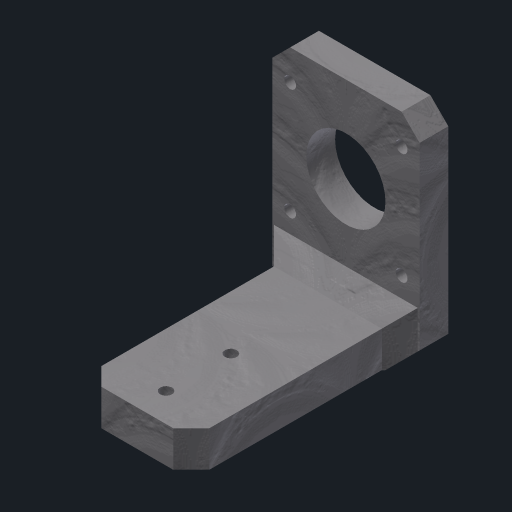
# Autodesk Inventor part: SOPORTE_NEMA_2
Saved by Autodesk Inventor 2024.3 (Build 283343000, 343)
## iProperties
Created: 2024-07-10
Part Number: SOPORTE_NEMA_2
Material: Steel, Mild, Welded
Document SubType Name: Modeling
Designer: Niler
Density: 7.85 g/cm^3
Appearance: Weld - Steel Mild
Author: Niler
Autodesk Inventor part; units mm, degrees
ref_plane "YZ Plane" through (0, 0, 0) normal (1, 0, 0) x (0, 1, 0)
ref_plane "XZ Plane" through (0, 0, 0) normal (0, 1, 0) x (-1, 0, 0)
ref_plane "XY Plane" through (0, 0, 0) normal (0, 0, 1) x (1, 0, 0)
sketch "Sketch1" plane through (0, 0, 0) normal (0, 1, 0) x (-1, 0, 0)
  line L0 (-15, 0) -> (15, 0)
  line L1 (15, 0) -> (15, -66)
  line L2 (15, -66) -> (-15, -66)
  line L3 (-15, -66) -> (-15, 0)
  circle A0 centre (0, -8) radius 1.65
  circle A1 centre (0, -26) radius 1.65
  point P0 (0, 0)
  point P1 (0, 0)
  dimension "d0" = 66
  dimension "d1" = 30
  dimension "d2" = 3.3
  dimension "d3" = 3.3
  dimension "d4" = 18
  dimension "d5" = 8
  constraints: 8 end point, 2 centre point, 2 coincident, 2 parallel, 1 horizontal, 1 midpoint, 1 perpendicular, 1 vertical alignment
  measures "d0" distance between parallel lines of L0 L2
  measures "d1" distance of L0.start L0.end
  measures "d2" diameter of A0
  measures "d3" diameter of A1
  measures "d4" distance of A1.centre A0.centre
  measures "d5" distance from line of L0 A0.centre
extrude "Extrusion1" add sketch "Sketch1" along normal blind 10
chamfer "Chamfer1" distance 5 angle 45 2 edges at (15, 5, 0) (-15, 5, 0)
sketch "Sketch2" plane through (15, 0, -66) normal (0, 0, -1) x (-1, 0, 0)
  line L0 (0, 0) -> (30, 0) projected
  line L1 (30, 0) -> (30, 10) projected
  line L2 (0, 10) -> (30, 10) projected
  line L3 (0, 0) -> (0, 10) projected
  line L4 (15, 0) -> (15, -14)
  line L5 (15, -14) -> (61, -14)
  line L6 (61, -14) -> (15, 36.0799)
  line L7 (15, 0) -> (15, 57.2033) construction
  circle A0 centre (15, 36.0799) radius 11
  line L8 (-0.5, 20.5799) -> (30.5, 20.5799) construction
  line L9 (30.5, 20.5799) -> (30.5, 51.5799) construction
  line L10 (30.5, 51.5799) -> (-0.5, 51.5799) construction
  line L11 (-0.5, 51.5799) -> (-0.5, 20.5799) construction
  line L12 (-0.5, 20.5799) -> (30.5, 51.5799) construction
  line L13 (30.5, 20.5799) -> (-0.5, 51.5799) construction
  circle A1 centre (-0.5, 51.5799) radius 1.65
  circle A2 centre (30.5, 51.5799) radius 1.65
  circle A3 centre (30.5, 20.5799) radius 1.65
  circle A4 centre (-0.5, 20.5799) radius 1.65
  line L14 (-5.5, 0) -> (35.5, 0)
  line L15 (35.5, 0) -> (35.5, 60)
  line L16 (35.5, 60) -> (-5.5, 60)
  line L17 (-5.5, 60) -> (-5.5, 0)
  dimension "d11" = 14
  dimension "d12" = 46
  dimension "d13" = 68
  dimension "d14" = 22
  dimension "d15" = 31
  dimension "d16" = 31
  dimension "d17" = 3.3
  dimension "d18" = 60
  dimension "d19" = 41
  constraints: 28 end point, 5 centre point, 5 coincident, 4 midpoint, 4 parallel, 3 equal radius, 3 perpendicular, 2 horizontal, 2 point on line, 1 vertical
  measures "d11" distance of L4.start L4.end
  measures "d12" distance of L4.end L5.end
  measures "d13" distance of L5.end L6.end
  measures "d14" diameter of A0
  measures "d15" distance of L10.end L9.end
  measures "d16" distance of L9.end L8.end
  measures "d17" diameter of A1
  measures "d18" distance of L14.end L15.end
  measures "d19" distance of L15.end L16.end
extrude "Extrusion2" add sketch "Sketch2" against normal blind 8 contours L14 L17 L16 L15 L1 L2 L3
chamfer "Chamfer2" distance 5 angle 45 7 edges at (20.5, 60, -62) (-20.5, 60, -62) (20.5, 0, -62) (15, 5, -58) (-15, 5, -58) (-20.5, 0, -62) (0, 10, -58)
body "Solid1"
